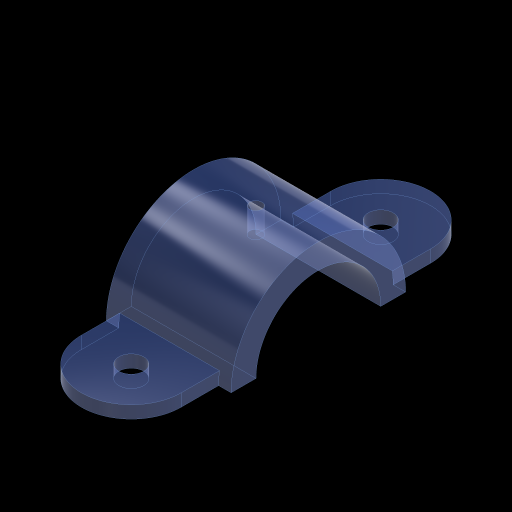
# Autodesk Inventor part: ANS8-TUT-BK
Saved by Autodesk Inventor 2024 (Build 280153000, 153)
## iProperties
Created: 2023-10-14
Part Number: ANS8-TUT-BK
Material: Water
Document SubType Name: Modeling
Designer: bennk
Mass: 119.569 g
Surface Area: 288.689 cm^2
Volume: 119.772 cm^3
Density: 0.9983 g/cm^3
Appearance: Tropical Blue
Author: bennk
Autodesk Inventor part; units mm, degrees
ref_plane "YZ Plane" through (0, 0, 0) normal (1, 0, 0) x (0, 1, 0)
ref_plane "XZ Plane" through (0, 0, 0) normal (0, 1, 0) x (-1, 0, 0)
ref_plane "XY Plane" through (0, 0, 0) normal (0, 0, 1) x (1, 0, 0)
sketch "Sketch1" plane through (0, 0, 0) normal (0, 1, 0) x (-1, 0, 0)
  line L0 (0, 88.9) -> (0, -88.9) construction
  line L1 (25.4, 63.5) -> (25.4, -63.5)
  line L2 (-25.4, -63.5) -> (-25.4, 63.5)
  arc A0 (25.4, 63.5) -> (-25.4, 63.5) centre (0, 63.5) ccw
  arc A1 (-25.4, -63.5) -> (25.4, -63.5) centre (0, -63.5) ccw
  circle A2 centre (0, 63.5) radius 6.35
  circle A3 centre (0, -63.5) radius 6.35
  point P0 (0, 0)
  point P1 (0, 0)
  dimension "d0" = 127
  dimension "d1" = 12.7
  dimension "d2" = 12.7
  dimension "d3" = 25.4
  constraints: 8 end point, 6 point on circle, 4 centre point, 4 tangent, 3 coincident, 2 point on line, 1 midpoint, 1 parallel, 1 vertical
  measures "d0" distance of A1.centre A0.centre
  measures "d1" diameter of A2
  measures "d2" diameter of A3
  measures "d3" radius of A1
extrude "BASE" add sketch "Sketch1" along normal blind 6.35
sketch "Sketch2" plane through (0, 0, 0) normal (1, 0, 0) x (0, 1, 0)
  arc A0 (0, -44.45) -> (0, 44.45) centre (0, 0) ccw
  arc A1 (0, -31.75) -> (0, 31.75) centre (0, 0) ccw
  line L0 (0, -63.5) -> (0, 63.5) projected
  dimension "d7" = 44.45
  dimension "d8" = 31.75
  constraints: 4 point on circle, 4 point on line, 2 centre point, 2 coincident
  measures "d7" radius of A0
  measures "d8" radius of A1
extrude "REMOVED CENTER OF BASE" cut sketch "Sketch2" along normal through all both and the other way through all contours L0 A1
extrude "ARCH" add sketch "Sketch2" along normal mid plane 63.5 contours L0 A1 A0
sketch "Sketch3" plane through (0, 0, 0) normal (0, 1, 0) x (-1, 0, 0)
  circle A0 centre (0, 0) radius 3.175
  dimension "d13" = 6.35
  constraints: 1 centre point, 1 coincident
  measures "d13" diameter of A0
extrude "TOPHOLE" cut sketch "Sketch3" along normal through all
equation "\"d2\" = d1"
body "Solid1"
